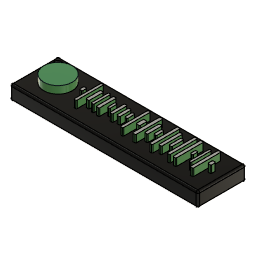
Spotify_Bars v3 (Autodesk Fusion 360 design; units mm, degrees)
Autodesk Fusion 360 part; units mm, degrees
sketch "Sketch1" plane through (0, 0, 0) normal (0, 0, 1) x (1, 0, 0)
  line L0 (0, 0) -> (50.8, 0)
  line L1 (50.8, 0) -> (50.8, 13.0624)
  line L2 (50.8, 13.0624) -> (0, 13.0624)
  line L3 (0, 13.0624) -> (0, 0)
  dimension "d1" = 50.8
  constraint horizontal L0
  constraint vertical L1
  constraint horizontal L2
  constraint vertical L3
  constraint coincident L0.start L3.end
  measures "d1" distance of L0.start L0.end
extrude "Extrude1" add sketch "Sketch1" along normal blind 4
sketch "Sketch2" plane through (0, 0, 4) normal (0, 0, 1) x (-1, 0, 0)
  line L0 (0, -13.0624) -> (0, 0)
  line L1 (0, 0) -> (-50.8, 0)
  line L2 (-50.8, 0) -> (-50.8, -13.0624)
  line L3 (-50.8, -13.0624) -> (0, -13.0624)
  line L4 (-12.7231, -7.3007) -> (-13.5424, -7.3007)
  line L5 (-13.5424, -7.3007) -> (-13.5424, -6.0226)
  line L6 (-13.5424, -6.0226) -> (-12.7231, -6.0226)
  line L7 (-12.7231, -6.0226) -> (-12.7231, -7.3007)
  constraint horizontal L4
  constraint vertical L5
  constraint horizontal L6
  constraint vertical L7
extrude "Extrude2" add sketch "Sketch2" along normal blind 2 contours L4 L5 L6 L7
sketch "Sketch3" plane through (0, 0, 4) normal (0, 0, 1) x (-1, 0, 0)
  line L0 (-12.7231, -6.0226) -> (-12.7231, -7.3007)
  line L1 (-12.7231, -7.3007) -> (-13.5424, -7.3007)
  line L2 (-13.5424, -7.3007) -> (-13.5424, -6.0226)
  line L3 (-13.5424, -6.0226) -> (-12.7231, -6.0226)
  line L4 (0, -13.0624) -> (0, 0)
  line L5 (0, 0) -> (-50.8, 0)
  line L6 (-50.8, 0) -> (-50.8, -13.0624)
  line L7 (-50.8, -13.0624) -> (0, -13.0624)
  line L8 (-14.2857, -10.434) -> (-15, -10.434)
  line L9 (-15, -10.434) -> (-15, -3)
  line L10 (-15, -3) -> (-14.2857, -3)
  line L11 (-14.2857, -3) -> (-14.2857, -10.434)
  constraint horizontal L8
  constraint vertical L9
  constraint horizontal L10
  constraint vertical L11
extrude "Extrude3" add sketch "Sketch3" along normal blind 2 contours L8 L9 L10 L11
sketch "Sketch4" plane through (0, 0, 4) normal (0, 0, 1) x (-1, 0, 0)
  line L0 (-14.2857, -3) -> (-14.2857, -10.434)
  line L1 (-14.2857, -10.434) -> (-15, -10.434)
  line L2 (-15, -10.434) -> (-15, -3)
  line L3 (-15, -3) -> (-14.2857, -3)
  line L4 (-12.7231, -6.0226) -> (-12.7231, -7.3007)
  line L5 (-12.7231, -7.3007) -> (-13.5424, -7.3007)
  line L6 (-13.5424, -7.3007) -> (-13.5424, -6.0226)
  line L7 (-13.5424, -6.0226) -> (-12.7231, -6.0226)
  line L8 (0, -13.0624) -> (0, 0)
  line L9 (0, 0) -> (-50.8, 0)
  line L10 (-50.8, 0) -> (-50.8, -13.0624)
  line L11 (-50.8, -13.0624) -> (0, -13.0624)
  line L12 (-15.8233, -8.6464) -> (-16.7081, -8.6464)
  line L13 (-16.7081, -8.6464) -> (-16.7081, -4.681)
  line L14 (-16.7081, -4.681) -> (-15.8233, -4.681)
  line L15 (-15.8233, -4.681) -> (-15.8233, -8.6464)
  constraint horizontal L12
  constraint vertical L13
  constraint horizontal L14
  constraint vertical L15
extrude "Extrude4" add sketch "Sketch4" along normal blind 2 contours L12 L13 L14 L15
sketch "Sketch5" plane through (0, 0, 4) normal (0, 0, 1) x (-1, 0, 0)
  line L0 (-15.8233, -4.681) -> (-15.8233, -8.6464)
  line L1 (-15.8233, -8.6464) -> (-16.7081, -8.6464)
  line L2 (-16.7081, -8.6464) -> (-16.7081, -4.681)
  line L3 (-16.7081, -4.681) -> (-15.8233, -4.681)
  line L4 (-14.2857, -3) -> (-14.2857, -10.434)
  line L5 (-14.2857, -10.434) -> (-15, -10.434)
  line L6 (-15, -10.434) -> (-15, -3)
  line L7 (-15, -3) -> (-14.2857, -3)
  line L8 (-12.7231, -6.0226) -> (-12.7231, -7.3007)
  line L9 (-12.7231, -7.3007) -> (-13.5424, -7.3007)
  line L10 (-13.5424, -7.3007) -> (-13.5424, -6.0226)
  line L11 (-13.5424, -6.0226) -> (-12.7231, -6.0226)
  line L12 (0, -13.0624) -> (0, 0)
  line L13 (0, 0) -> (-50.8, 0)
  line L14 (-50.8, 0) -> (-50.8, -13.0624)
  line L15 (-50.8, -13.0624) -> (0, -13.0624)
  line L16 (-17.5123, -9.1117) -> (-18.2005, -9.1117)
  line L17 (-18.2005, -9.1117) -> (-18.2005, -4.3925)
  line L18 (-18.2005, -4.3925) -> (-17.5123, -4.3925)
  line L19 (-17.5123, -4.3925) -> (-17.5123, -9.1117)
  constraint horizontal L16
  constraint vertical L17
  constraint horizontal L18
  constraint vertical L19
extrude "Extrude5" add sketch "Sketch5" along normal blind 2 contours L16 L17 L18 L19
sketch "Sketch6" plane through (0, 0, 4) normal (0, 0, 1) x (-1, 0, 0)
  line L0 (-17.5123, -4.3925) -> (-17.5123, -9.1117)
  line L1 (-17.5123, -9.1117) -> (-18.2005, -9.1117)
  line L2 (-18.2005, -9.1117) -> (-18.2005, -4.3925)
  line L3 (-18.2005, -4.3925) -> (-17.5123, -4.3925)
  line L4 (-15.8233, -4.681) -> (-15.8233, -8.6464)
  line L5 (-15.8233, -8.6464) -> (-16.7081, -8.6464)
  line L6 (-16.7081, -8.6464) -> (-16.7081, -4.681)
  line L7 (-16.7081, -4.681) -> (-15.8233, -4.681)
  line L8 (-14.2857, -3) -> (-14.2857, -10.434)
  line L9 (-14.2857, -10.434) -> (-15, -10.434)
  line L10 (-15, -10.434) -> (-15, -3)
  line L11 (-15, -3) -> (-14.2857, -3)
  line L12 (-12.7231, -6.0226) -> (-12.7231, -7.3007)
  line L13 (-12.7231, -7.3007) -> (-13.5424, -7.3007)
  line L14 (-13.5424, -7.3007) -> (-13.5424, -6.0226)
  line L15 (-13.5424, -6.0226) -> (-12.7231, -6.0226)
  line L16 (0, -13.0624) -> (0, 0)
  line L17 (0, 0) -> (-50.8, 0)
  line L18 (-50.8, 0) -> (-50.8, -13.0624)
  line L19 (-50.8, -13.0624) -> (0, -13.0624)
  line L20 (-19, -9) -> (-19.8456, -9)
  line L21 (-19.8456, -9) -> (-19.8456, -4.261)
  line L22 (-19.8456, -4.261) -> (-19, -4.261)
  line L23 (-19, -4.261) -> (-19, -9)
  line L24 (-20.6977, -7.7349) -> (-21.3531, -7.7349)
  line L25 (-21.3531, -7.7349) -> (-21.3531, -5.6047)
  line L26 (-21.3531, -5.6047) -> (-20.6977, -5.6047)
  line L27 (-20.6977, -5.6047) -> (-20.6977, -7.7349)
  line L28 (-22.2708, -8.718) -> (-23.0573, -8.718)
  line L29 (-23.0573, -8.718) -> (-23.0573, -4.687)
  line L30 (-23.0573, -4.687) -> (-22.2708, -4.687)
  line L31 (-22.2708, -4.687) -> (-22.2708, -8.718)
  line L32 (-23.8111, -8.2592) -> (-24.6304, -8.2592)
  line L33 (-24.6304, -8.2592) -> (-24.6304, -5.0475)
  line L34 (-24.6304, -5.0475) -> (-23.8111, -5.0475)
  line L35 (-23.8111, -5.0475) -> (-23.8111, -8.2592)
  line L36 (-25.3514, -7.7349) -> (-26.1051, -7.7349)
  line L37 (-26.1051, -7.7349) -> (-26.1051, -5.6374)
  line L38 (-26.1051, -5.6374) -> (-25.3514, -5.6374)
  line L39 (-25.3514, -5.6374) -> (-25.3514, -7.7349)
  line L40 (-26.9572, -10.3567) -> (-27.711, -10.3567)
  line L41 (-27.711, -10.3567) -> (-27.711, -2.8845)
  line L42 (-27.711, -2.8845) -> (-26.9572, -2.8845)
  line L43 (-26.9572, -2.8845) -> (-26.9572, -10.3567)
  line L44 (-28.432, -7.7021) -> (-29.4479, -7.7021)
  line L45 (-29.4479, -7.7021) -> (-29.4479, -5.6374)
  line L46 (-29.4479, -5.6374) -> (-28.432, -5.6374)
  line L47 (-28.432, -5.6374) -> (-28.432, -7.7021)
  line L48 (-30.1034, -10.3894) -> (-31, -10.3894)
  line L49 (-31, -10.3894) -> (-31, -3)
  line L50 (-31, -3) -> (-30.1034, -3)
  line L51 (-30.1034, -3) -> (-30.1034, -10.3894)
  line L52 (-31.6437, -8.718) -> (-32.4957, -8.718)
  line L53 (-32.4957, -8.718) -> (-32.4957, -4.687)
  line L54 (-32.4957, -4.687) -> (-31.6437, -4.687)
  line L55 (-31.6437, -4.687) -> (-31.6437, -8.718)
  line L56 (-33.2495, -7.7349) -> (-34.0033, -7.7349)
  line L57 (-34.0033, -7.7349) -> (-34.0033, -5.5719)
  line L58 (-34.0033, -5.5719) -> (-33.2495, -5.5719)
  line L59 (-33.2495, -5.5719) -> (-33.2495, -7.7349)
  line L60 (-34.7898, -10.4877) -> (-35.6091, -10.4877)
  line L61 (-35.6091, -10.4877) -> (-35.6091, -2.8845)
  line L62 (-35.6091, -2.8845) -> (-34.7898, -2.8845)
  line L63 (-34.7898, -2.8845) -> (-34.7898, -10.4877)
  line L64 (-36.3957, -9.5373) -> (-37.215, -9.5373)
  line L65 (-37.215, -9.5373) -> (-37.215, -3.7694)
  line L66 (-37.215, -3.7694) -> (-36.3957, -3.7694)
  line L67 (-36.3957, -3.7694) -> (-36.3957, -9.5373)
  line L68 (-37.9032, -8.3575) -> (-38.6897, -8.3575)
  line L69 (-38.6897, -8.3575) -> (-38.6897, -5.0475)
  line L70 (-38.6897, -5.0475) -> (-37.9032, -5.0475)
  line L71 (-37.9032, -5.0475) -> (-37.9032, -8.3575)
  line L72 (-39.509, -10.455) -> (-40.2956, -10.455)
  line L73 (-40.2956, -10.455) -> (-40.2956, -2.9501)
  line L74 (-40.2956, -2.9501) -> (-39.509, -2.9501)
  line L75 (-39.509, -2.9501) -> (-39.509, -10.455)
  line L76 (-41.0821, -10.455) -> (-41.9342, -10.455)
  line L77 (-41.9342, -10.455) -> (-41.9342, -2.9501)
  line L78 (-41.9342, -2.9501) -> (-41.0821, -2.9501)
  line L79 (-41.0821, -2.9501) -> (-41.0821, -10.455)
  line L80 (-42.7535, -7.4399) -> (-43.4417, -7.4399)
  line L81 (-43.4417, -7.4399) -> (-43.4417, -5.9979)
  line L82 (-43.4417, -5.9979) -> (-42.7535, -5.9979)
  line L83 (-42.7535, -5.9979) -> (-42.7535, -7.4399)
  line L84 (-44.3594, -9.5701) -> (-45, -9.5701)
  line L85 (-45, -9.5701) -> (-45, -4)
  line L86 (-45, -4) -> (-44.3594, -4)
  line L87 (-44.3594, -4) -> (-44.3594, -9.5701)
  line L88 (-45.8669, -10.4877) -> (-46.6534, -10.4877)
  line L89 (-46.6534, -10.4877) -> (-46.6534, -2.9501)
  line L90 (-46.6534, -2.9501) -> (-45.8669, -2.9501)
  line L91 (-45.8669, -2.9501) -> (-45.8669, -10.4877)
  line L92 (-47.44, -7.3744) -> (-48.2921, -7.3744)
  line L93 (-48.2921, -7.3744) -> (-48.2921, -5.9979)
  line L94 (-48.2921, -5.9979) -> (-47.44, -5.9979)
  line L95 (-47.44, -5.9979) -> (-47.44, -7.3744)
  constraint horizontal L20
  constraint vertical L21
  constraint horizontal L22
  constraint vertical L23
  constraint horizontal L24
  constraint vertical L25
  constraint horizontal L26
  constraint vertical L27
  constraint horizontal L28
  constraint vertical L29
  constraint horizontal L30
  constraint vertical L31
  constraint horizontal L32
  constraint vertical L33
  constraint horizontal L34
  constraint vertical L35
  constraint horizontal L36
  constraint vertical L37
  constraint horizontal L38
  constraint vertical L39
  constraint horizontal L40
  constraint vertical L41
  constraint horizontal L42
  constraint vertical L43
  constraint horizontal L44
  constraint vertical L45
  constraint horizontal L46
  constraint vertical L47
  constraint horizontal L48
  constraint vertical L49
  constraint horizontal L50
  constraint vertical L51
  constraint horizontal L52
  constraint vertical L53
  constraint horizontal L54
  constraint vertical L55
  constraint horizontal L56
  constraint vertical L57
  constraint horizontal L58
  constraint vertical L59
  constraint horizontal L60
  constraint vertical L61
  constraint horizontal L62
  constraint vertical L63
  constraint horizontal L64
  constraint vertical L65
  constraint horizontal L66
  constraint vertical L67
  constraint horizontal L68
  constraint vertical L69
  constraint horizontal L70
  constraint vertical L71
  constraint horizontal L72
  constraint vertical L73
  constraint horizontal L74
  constraint vertical L75
  constraint horizontal L76
  constraint vertical L77
  constraint horizontal L78
  constraint vertical L79
  constraint horizontal L80
  constraint vertical L81
  constraint horizontal L82
  constraint vertical L83
  constraint horizontal L84
  constraint vertical L85
  constraint horizontal L86
  constraint vertical L87
  constraint horizontal L88
  constraint vertical L89
  constraint horizontal L90
  constraint vertical L91
  constraint horizontal L92
  constraint vertical L93
  constraint horizontal L94
  constraint vertical L95
extrude "Extrude6" add sketch "Sketch6" along normal blind 2 contours L20 L21 L22 L23 | L24 L25 L26 L27 | L28 L29 L30 L31 | L32 L33 L34 L35 | L36 L37 L38 L39 | L40 L41 L42 L43 | L44 L45 L46 L47 | L48 L49 L50 L51 | L52 L53 L54 L55 | L56 L57 L58 L59 | L60 L61 L62 L63 | L64 L65 L66 L67 | L68 L69 L70 L71 | L72 L73 L74 L75 | L76 L77 L78 L79 | L80 L81 L82 L83 | L84 L85 L86 L87
sketch "Sketch7" plane through (0, 0, 4) normal (0, 0, 1) x (-1, 0, 0)
  line L0 (-19, -4.261) -> (-19, -9)
  line L1 (-19, -9) -> (-19.8456, -9)
  line L2 (-19.8456, -9) -> (-19.8456, -4.261)
  line L3 (-19.8456, -4.261) -> (-19, -4.261)
  line L4 (-25.3514, -5.6374) -> (-25.3514, -7.7349)
  line L5 (-25.3514, -7.7349) -> (-26.1051, -7.7349)
  line L6 (-26.1051, -7.7349) -> (-26.1051, -5.6374)
  line L7 (-26.1051, -5.6374) -> (-25.3514, -5.6374)
  line L8 (-31.6437, -4.687) -> (-31.6437, -8.718)
  line L9 (-31.6437, -8.718) -> (-32.4957, -8.718)
  line L10 (-32.4957, -8.718) -> (-32.4957, -4.687)
  line L11 (-32.4957, -4.687) -> (-31.6437, -4.687)
  line L12 (-37.9032, -5.0475) -> (-37.9032, -8.3575)
  line L13 (-37.9032, -8.3575) -> (-38.6897, -8.3575)
  line L14 (-38.6897, -8.3575) -> (-38.6897, -5.0475)
  line L15 (-38.6897, -5.0475) -> (-37.9032, -5.0475)
  line L16 (-44.3594, -4) -> (-44.3594, -9.5701)
  line L17 (-44.3594, -9.5701) -> (-45, -9.5701)
  line L18 (-45, -9.5701) -> (-45, -4)
  line L19 (-45, -4) -> (-44.3594, -4)
  line L20 (-39.509, -2.9501) -> (-39.509, -10.455)
  line L21 (-39.509, -10.455) -> (-40.2956, -10.455)
  line L22 (-40.2956, -10.455) -> (-40.2956, -2.9501)
  line L23 (-40.2956, -2.9501) -> (-39.509, -2.9501)
  line L24 (-33.2495, -5.5719) -> (-33.2495, -7.7349)
  line L25 (-33.2495, -7.7349) -> (-34.0033, -7.7349)
  line L26 (-34.0033, -7.7349) -> (-34.0033, -5.5719)
  line L27 (-34.0033, -5.5719) -> (-33.2495, -5.5719)
  line L28 (-26.9572, -2.8845) -> (-26.9572, -10.3567)
  line L29 (-26.9572, -10.3567) -> (-27.711, -10.3567)
  line L30 (-27.711, -10.3567) -> (-27.711, -2.8845)
  line L31 (-27.711, -2.8845) -> (-26.9572, -2.8845)
  line L32 (-20.6977, -5.6047) -> (-20.6977, -7.7349)
  line L33 (-20.6977, -7.7349) -> (-21.3531, -7.7349)
  line L34 (-21.3531, -7.7349) -> (-21.3531, -5.6047)
  line L35 (-21.3531, -5.6047) -> (-20.6977, -5.6047)
  line L36 (-23.8111, -5.0475) -> (-23.8111, -8.2592)
  line L37 (-23.8111, -8.2592) -> (-24.6304, -8.2592)
  line L38 (-24.6304, -8.2592) -> (-24.6304, -5.0475)
  line L39 (-24.6304, -5.0475) -> (-23.8111, -5.0475)
  line L40 (-30.1034, -3) -> (-30.1034, -10.3894)
  line L41 (-30.1034, -10.3894) -> (-31, -10.3894)
  line L42 (-31, -10.3894) -> (-31, -3)
  line L43 (-31, -3) -> (-30.1034, -3)
  line L44 (-36.3957, -3.7694) -> (-36.3957, -9.5373)
  line L45 (-36.3957, -9.5373) -> (-37.215, -9.5373)
  line L46 (-37.215, -9.5373) -> (-37.215, -3.7694)
  line L47 (-37.215, -3.7694) -> (-36.3957, -3.7694)
  line L48 (-42.7535, -5.9979) -> (-42.7535, -7.4399)
  line L49 (-42.7535, -7.4399) -> (-43.4417, -7.4399)
  line L50 (-43.4417, -7.4399) -> (-43.4417, -5.9979)
  line L51 (-43.4417, -5.9979) -> (-42.7535, -5.9979)
  line L52 (-41.0821, -2.9501) -> (-41.0821, -10.455)
  line L53 (-41.0821, -10.455) -> (-41.9342, -10.455)
  line L54 (-41.9342, -10.455) -> (-41.9342, -2.9501)
  line L55 (-41.9342, -2.9501) -> (-41.0821, -2.9501)
  line L56 (-34.7898, -2.8845) -> (-34.7898, -10.4877)
  line L57 (-34.7898, -10.4877) -> (-35.6091, -10.4877)
  line L58 (-35.6091, -10.4877) -> (-35.6091, -2.8845)
  line L59 (-35.6091, -2.8845) -> (-34.7898, -2.8845)
  line L60 (-28.432, -5.6374) -> (-28.432, -7.7021)
  line L61 (-28.432, -7.7021) -> (-29.4479, -7.7021)
  line L62 (-29.4479, -7.7021) -> (-29.4479, -5.6374)
  line L63 (-29.4479, -5.6374) -> (-28.432, -5.6374)
  line L64 (-22.2708, -4.687) -> (-22.2708, -8.718)
  line L65 (-22.2708, -8.718) -> (-23.0573, -8.718)
  line L66 (-23.0573, -8.718) -> (-23.0573, -4.687)
  line L67 (-23.0573, -4.687) -> (-22.2708, -4.687)
  line L68 (-17.5123, -4.3925) -> (-17.5123, -9.1117)
  line L69 (-17.5123, -9.1117) -> (-18.2005, -9.1117)
  line L70 (-18.2005, -9.1117) -> (-18.2005, -4.3925)
  line L71 (-18.2005, -4.3925) -> (-17.5123, -4.3925)
  line L72 (-15.8233, -4.681) -> (-15.8233, -8.6464)
  line L73 (-15.8233, -8.6464) -> (-16.7081, -8.6464)
  line L74 (-16.7081, -8.6464) -> (-16.7081, -4.681)
  line L75 (-16.7081, -4.681) -> (-15.8233, -4.681)
  line L76 (-14.2857, -3) -> (-14.2857, -10.434)
  line L77 (-14.2857, -10.434) -> (-15, -10.434)
  line L78 (-15, -10.434) -> (-15, -3)
  line L79 (-15, -3) -> (-14.2857, -3)
  line L80 (-12.7231, -6.0226) -> (-12.7231, -7.3007)
  line L81 (-12.7231, -7.3007) -> (-13.5424, -7.3007)
  line L82 (-13.5424, -7.3007) -> (-13.5424, -6.0226)
  line L83 (-13.5424, -6.0226) -> (-12.7231, -6.0226)
  line L84 (0, -13.0624) -> (0, 0)
  line L85 (0, 0) -> (-50.8, 0)
  line L86 (-50.8, 0) -> (-50.8, -13.0624)
  line L87 (-50.8, -13.0624) -> (0, -13.0624)
  line L88 (-45.7946, -10.487) -> (-46.614, -10.487)
  line L89 (-46.614, -10.487) -> (-46.614, -2.8838)
  line L90 (-46.614, -2.8838) -> (-45.7946, -2.8838)
  line L91 (-45.7946, -2.8838) -> (-45.7946, -10.487)
  line L92 (-47.4333, -7.3408) -> (-48.3181, -7.3408)
  line L93 (-48.3181, -7.3408) -> (-48.3181, -6.0299)
  line L94 (-48.3181, -6.0299) -> (-47.4333, -6.0299)
  line L95 (-47.4333, -6.0299) -> (-47.4333, -7.3408)
  constraint horizontal L88
  constraint vertical L89
  constraint horizontal L90
  constraint vertical L91
  constraint horizontal L92
  constraint vertical L93
  constraint horizontal L94
  constraint vertical L95
extrude "Extrude7" add sketch "Sketch7" along normal blind 2 contours L88 L89 L90 L91 | L92 L93 L94 L95
fillet "Fillet1" radius 0.2 3 edges at (12.7231, 6.0226, 5) (12.7231, 7.3007, 5) (13.5424, 6.0226, 5)
fillet "Fillet2" radius 0.2 45 edges at (14.2857, 10.434, 5) (15, 10.434, 5) (15, 3, 5) (15.8233, 8.6464, 5) (16.7081, 8.6464, 5) (17.5123, 9.1117, 5) (16.7081, 4.681, 5) (15.8233, 4.681, 5) (14.2857, 3, 5) (13.5424, 7.3007, 5) (17.5123, 4.3925, 5) (18.2005, 9.1117, 5) (18.2005, 4.3925, 5) (19, 9, 5) (19.8456, 9, 5) (19, 4.261, 5) (19.8456, 4.261, 5) (20.6977, 7.7349, 5) (20.6977, 5.6047, 5) (21.3531, 7.7349, 5) (21.3531, 5.6047, 5) (22.2708, 8.718, 5) (23.0573, 8.718, 5) (22.2708, 4.687, 5) (23.0573, 4.687, 5) (23.8111, 8.2592, 5) (23.8111, 5.0475, 5) (24.6304, 8.2592, 5) (24.6304, 5.0475, 5) (25.3514, 7.7349, 5) (25.3514, 5.6374, 5) (26.1051, 7.7349, 5) (26.1051, 5.6374, 5) (26.9572, 10.3567, 5) (27.711, 10.3567, 5) (26.9572, 2.8845, 5) (27.711, 2.8845, 5) (28.432, 7.7021, 5) (28.432, 5.6374, 5) (29.4479, 7.7021, 5) (29.4479, 5.6374, 5) (30.1034, 10.3894, 5) (30.1034, 3, 5) (31, 10.3894, 5) (31.6437, 8.718, 5)
fillet "Fillet3" radius 0.2 44 edges at (31.6437, 4.687, 5) (31, 3, 5) (32.4957, 4.687, 5) (32.4957, 8.718, 5) (33.2495, 5.5719, 5) (33.2495, 7.7349, 5) (34.0033, 7.7349, 5) (34.0033, 5.5719, 5) (34.7898, 10.4877, 5) (35.6091, 10.4877, 5) (34.7898, 2.8845, 5) (35.6091, 2.8845, 5) (36.3957, 9.5373, 5) (36.3957, 3.7694, 5) (37.215, 9.5373, 5) (37.215, 3.7694, 5) (37.9032, 8.3575, 5) (37.9032, 5.0475, 5) (38.6897, 8.3575, 5) (38.6897, 5.0475, 5) (39.509, 10.455, 5) (39.509, 2.9501, 5) (40.2956, 10.455, 5) (40.2956, 2.9501, 5) (41.0821, 10.455, 5) (41.0821, 2.9501, 5) (41.9342, 10.455, 5) (41.9342, 2.9501, 5) (42.7535, 7.4399, 5) (42.7535, 5.9979, 5) (43.4417, 5.9979, 5) (43.4417, 7.4399, 5) (44.3594, 9.5701, 5) (45, 9.5701, 5) (44.3594, 4, 5) (45, 4, 5) (45.7946, 10.487, 5) (45.7946, 2.8838, 5) (46.614, 10.487, 5) (46.614, 2.8838, 5) (47.4333, 7.3408, 5) (47.4333, 6.0299, 5) (48.3181, 7.3408, 5) (48.3181, 6.0299, 5)
sketch "Sketch8" plane through (0, 0, 4) normal (0, 0, 1) x (-1, 0, 0)
  line L0 (-47.4333, -6.2299) -> (-47.4333, -7.1408)
  arc A0 (-47.6333, -7.3408) -> (-47.4333, -7.1408) centre (-47.6333, -7.1408) ccw
  line L1 (-47.6333, -7.3408) -> (-48.1181, -7.3408)
  arc A1 (-48.3181, -7.1408) -> (-48.1181, -7.3408) centre (-48.1181, -7.1408) ccw
  line L2 (-48.3181, -7.1408) -> (-48.3181, -6.2299)
  arc A2 (-48.1181, -6.0299) -> (-48.3181, -6.2299) centre (-48.1181, -6.2299) ccw
  line L3 (-48.1181, -6.0299) -> (-47.6333, -6.0299)
  arc A3 (-47.4333, -6.2299) -> (-47.6333, -6.0299) centre (-47.6333, -6.2299) ccw
  line L4 (-45.7946, -3.0838) -> (-45.7946, -10.287)
  arc A4 (-45.9946, -10.487) -> (-45.7946, -10.287) centre (-45.9946, -10.287) ccw
  line L5 (-45.9946, -10.487) -> (-46.414, -10.487)
  arc A5 (-46.614, -10.287) -> (-46.414, -10.487) centre (-46.414, -10.287) ccw
  line L6 (-46.614, -10.287) -> (-46.614, -3.0838)
  arc A6 (-46.414, -2.8838) -> (-46.614, -3.0838) centre (-46.414, -3.0838) ccw
  line L7 (-46.414, -2.8838) -> (-45.9946, -2.8838)
  arc A7 (-45.7946, -3.0838) -> (-45.9946, -2.8838) centre (-45.9946, -3.0838) ccw
  line L8 (-19, -4.461) -> (-19, -8.8)
  arc A8 (-19.2, -9) -> (-19, -8.8) centre (-19.2, -8.8) ccw
  line L9 (-19.2, -9) -> (-19.6456, -9)
  arc A9 (-19.8456, -8.8) -> (-19.6456, -9) centre (-19.6456, -8.8) ccw
  line L10 (-19.8456, -8.8) -> (-19.8456, -4.461)
  arc A10 (-19.6456, -4.261) -> (-19.8456, -4.461) centre (-19.6456, -4.461) ccw
  line L11 (-19.6456, -4.261) -> (-19.2, -4.261)
  arc A11 (-19, -4.461) -> (-19.2, -4.261) centre (-19.2, -4.461) ccw
  line L12 (-25.3514, -5.8374) -> (-25.3514, -7.5349)
  arc A12 (-25.5514, -7.7349) -> (-25.3514, -7.5349) centre (-25.5514, -7.5349) ccw
  line L13 (-25.5514, -7.7349) -> (-25.9051, -7.7349)
  arc A13 (-26.1051, -7.5349) -> (-25.9051, -7.7349) centre (-25.9051, -7.5349) ccw
  line L14 (-26.1051, -7.5349) -> (-26.1051, -5.8374)
  arc A14 (-25.9051, -5.6374) -> (-26.1051, -5.8374) centre (-25.9051, -5.8374) ccw
  line L15 (-25.9051, -5.6374) -> (-25.5514, -5.6374)
  arc A15 (-25.3514, -5.8374) -> (-25.5514, -5.6374) centre (-25.5514, -5.8374) ccw
  line L16 (-31.6437, -4.887) -> (-31.6437, -8.518)
  arc A16 (-31.8437, -8.718) -> (-31.6437, -8.518) centre (-31.8437, -8.518) ccw
  line L17 (-31.8437, -8.718) -> (-32.2957, -8.718)
  arc A17 (-32.4957, -8.518) -> (-32.2957, -8.718) centre (-32.2957, -8.518) ccw
  line L18 (-32.4957, -8.518) -> (-32.4957, -4.887)
  arc A18 (-32.2957, -4.687) -> (-32.4957, -4.887) centre (-32.2957, -4.887) ccw
  line L19 (-32.2957, -4.687) -> (-31.8437, -4.687)
  arc A19 (-31.6437, -4.887) -> (-31.8437, -4.687) centre (-31.8437, -4.887) ccw
  line L20 (-37.9032, -5.2475) -> (-37.9032, -8.1575)
  arc A20 (-38.1032, -8.3575) -> (-37.9032, -8.1575) centre (-38.1032, -8.1575) ccw
  line L21 (-38.1032, -8.3575) -> (-38.4897, -8.3575)
  arc A21 (-38.6897, -8.1575) -> (-38.4897, -8.3575) centre (-38.4897, -8.1575) ccw
  line L22 (-38.6897, -8.1575) -> (-38.6897, -5.2475)
  arc A22 (-38.4897, -5.0475) -> (-38.6897, -5.2475) centre (-38.4897, -5.2475) ccw
  line L23 (-38.4897, -5.0475) -> (-38.1032, -5.0475)
  arc A23 (-37.9032, -5.2475) -> (-38.1032, -5.0475) centre (-38.1032, -5.2475) ccw
  line L24 (-44.3594, -4.2) -> (-44.3594, -9.3701)
  arc A24 (-44.5594, -9.5701) -> (-44.3594, -9.3701) centre (-44.5594, -9.3701) ccw
  line L25 (-44.5594, -9.5701) -> (-44.8, -9.5701)
  arc A25 (-45, -9.3701) -> (-44.8, -9.5701) centre (-44.8, -9.3701) ccw
  line L26 (-45, -9.3701) -> (-45, -4.2)
  arc A26 (-44.8, -4) -> (-45, -4.2) centre (-44.8, -4.2) ccw
  line L27 (-44.8, -4) -> (-44.5594, -4)
  arc A27 (-44.3594, -4.2) -> (-44.5594, -4) centre (-44.5594, -4.2) ccw
  line L28 (-39.509, -3.1501) -> (-39.509, -10.255)
  arc A28 (-39.709, -10.455) -> (-39.509, -10.255) centre (-39.709, -10.255) ccw
  line L29 (-39.709, -10.455) -> (-40.0956, -10.455)
  arc A29 (-40.2956, -10.255) -> (-40.0956, -10.455) centre (-40.0956, -10.255) ccw
  line L30 (-40.2956, -10.255) -> (-40.2956, -3.1501)
  arc A30 (-40.0956, -2.9501) -> (-40.2956, -3.1501) centre (-40.0956, -3.1501) ccw
  line L31 (-40.0956, -2.9501) -> (-39.709, -2.9501)
  arc A31 (-39.509, -3.1501) -> (-39.709, -2.9501) centre (-39.709, -3.1501) ccw
  line L32 (-33.2495, -5.7719) -> (-33.2495, -7.5349)
  arc A32 (-33.4495, -7.7349) -> (-33.2495, -7.5349) centre (-33.4495, -7.5349) ccw
  line L33 (-33.4495, -7.7349) -> (-33.8033, -7.7349)
  arc A33 (-34.0033, -7.5349) -> (-33.8033, -7.7349) centre (-33.8033, -7.5349) ccw
  line L34 (-34.0033, -7.5349) -> (-34.0033, -5.7719)
  arc A34 (-33.8033, -5.5719) -> (-34.0033, -5.7719) centre (-33.8033, -5.7719) ccw
  line L35 (-33.8033, -5.5719) -> (-33.4495, -5.5719)
  arc A35 (-33.2495, -5.7719) -> (-33.4495, -5.5719) centre (-33.4495, -5.7719) ccw
  line L36 (-26.9572, -3.0845) -> (-26.9572, -10.1567)
  arc A36 (-27.1572, -10.3567) -> (-26.9572, -10.1567) centre (-27.1572, -10.1567) ccw
  line L37 (-27.1572, -10.3567) -> (-27.511, -10.3567)
  arc A37 (-27.711, -10.1567) -> (-27.511, -10.3567) centre (-27.511, -10.1567) ccw
  line L38 (-27.711, -10.1567) -> (-27.711, -3.0845)
  arc A38 (-27.511, -2.8845) -> (-27.711, -3.0845) centre (-27.511, -3.0845) ccw
  line L39 (-27.511, -2.8845) -> (-27.1572, -2.8845)
  arc A39 (-26.9572, -3.0845) -> (-27.1572, -2.8845) centre (-27.1572, -3.0845) ccw
  line L40 (-20.6977, -5.8047) -> (-20.6977, -7.5349)
  arc A40 (-20.8977, -7.7349) -> (-20.6977, -7.5349) centre (-20.8977, -7.5349) ccw
  line L41 (-20.8977, -7.7349) -> (-21.1531, -7.7349)
  arc A41 (-21.3531, -7.5349) -> (-21.1531, -7.7349) centre (-21.1531, -7.5349) ccw
  line L42 (-21.3531, -7.5349) -> (-21.3531, -5.8047)
  arc A42 (-21.1531, -5.6047) -> (-21.3531, -5.8047) centre (-21.1531, -5.8047) ccw
  line L43 (-21.1531, -5.6047) -> (-20.8977, -5.6047)
  arc A43 (-20.6977, -5.8047) -> (-20.8977, -5.6047) centre (-20.8977, -5.8047) ccw
  line L44 (-23.8111, -5.2475) -> (-23.8111, -8.0592)
  arc A44 (-24.0111, -8.2592) -> (-23.8111, -8.0592) centre (-24.0111, -8.0592) ccw
  line L45 (-24.0111, -8.2592) -> (-24.4304, -8.2592)
  arc A45 (-24.6304, -8.0592) -> (-24.4304, -8.2592) centre (-24.4304, -8.0592) ccw
  line L46 (-24.6304, -8.0592) -> (-24.6304, -5.2475)
  arc A46 (-24.4304, -5.0475) -> (-24.6304, -5.2475) centre (-24.4304, -5.2475) ccw
  line L47 (-24.4304, -5.0475) -> (-24.0111, -5.0475)
  arc A47 (-23.8111, -5.2475) -> (-24.0111, -5.0475) centre (-24.0111, -5.2475) ccw
  line L48 (-30.1034, -3.2) -> (-30.1034, -10.1894)
  arc A48 (-30.3034, -10.3894) -> (-30.1034, -10.1894) centre (-30.3034, -10.1894) ccw
  line L49 (-30.3034, -10.3894) -> (-30.8, -10.3894)
  arc A49 (-31, -10.1894) -> (-30.8, -10.3894) centre (-30.8, -10.1894) ccw
  line L50 (-31, -10.1894) -> (-31, -3.2)
  arc A50 (-30.8, -3) -> (-31, -3.2) centre (-30.8, -3.2) ccw
  line L51 (-30.8, -3) -> (-30.3034, -3)
  arc A51 (-30.1034, -3.2) -> (-30.3034, -3) centre (-30.3034, -3.2) ccw
  line L52 (-36.3957, -3.9694) -> (-36.3957, -9.3373)
  arc A52 (-36.5957, -9.5373) -> (-36.3957, -9.3373) centre (-36.5957, -9.3373) ccw
  line L53 (-36.5957, -9.5373) -> (-37.015, -9.5373)
  arc A53 (-37.215, -9.3373) -> (-37.015, -9.5373) centre (-37.015, -9.3373) ccw
  line L54 (-37.215, -9.3373) -> (-37.215, -3.9694)
  arc A54 (-37.015, -3.7694) -> (-37.215, -3.9694) centre (-37.015, -3.9694) ccw
  line L55 (-37.015, -3.7694) -> (-36.5957, -3.7694)
  arc A55 (-36.3957, -3.9694) -> (-36.5957, -3.7694) centre (-36.5957, -3.9694) ccw
  line L56 (-42.7535, -6.1979) -> (-42.7535, -7.2399)
  arc A56 (-42.9535, -7.4399) -> (-42.7535, -7.2399) centre (-42.9535, -7.2399) ccw
  line L57 (-42.9535, -7.4399) -> (-43.2417, -7.4399)
  arc A57 (-43.4417, -7.2399) -> (-43.2417, -7.4399) centre (-43.2417, -7.2399) ccw
  line L58 (-43.4417, -7.2399) -> (-43.4417, -6.1979)
  arc A58 (-43.2417, -5.9979) -> (-43.4417, -6.1979) centre (-43.2417, -6.1979) ccw
  line L59 (-43.2417, -5.9979) -> (-42.9535, -5.9979)
  arc A59 (-42.7535, -6.1979) -> (-42.9535, -5.9979) centre (-42.9535, -6.1979) ccw
  line L60 (-41.0821, -3.1501) -> (-41.0821, -10.255)
  arc A60 (-41.2821, -10.455) -> (-41.0821, -10.255) centre (-41.2821, -10.255) ccw
  line L61 (-41.2821, -10.455) -> (-41.7342, -10.455)
  arc A61 (-41.9342, -10.255) -> (-41.7342, -10.455) centre (-41.7342, -10.255) ccw
  line L62 (-41.9342, -10.255) -> (-41.9342, -3.1501)
  arc A62 (-41.7342, -2.9501) -> (-41.9342, -3.1501) centre (-41.7342, -3.1501) ccw
  line L63 (-41.7342, -2.9501) -> (-41.2821, -2.9501)
  arc A63 (-41.0821, -3.1501) -> (-41.2821, -2.9501) centre (-41.2821, -3.1501) ccw
  line L64 (-34.7898, -3.0845) -> (-34.7898, -10.2877)
  arc A64 (-34.9898, -10.4877) -> (-34.7898, -10.2877) centre (-34.9898, -10.2877) ccw
  line L65 (-34.9898, -10.4877) -> (-35.4091, -10.4877)
  arc A65 (-35.6091, -10.2877) -> (-35.4091, -10.4877) centre (-35.4091, -10.2877) ccw
  line L66 (-35.6091, -10.2877) -> (-35.6091, -3.0845)
  arc A66 (-35.4091, -2.8845) -> (-35.6091, -3.0845) centre (-35.4091, -3.0845) ccw
  line L67 (-35.4091, -2.8845) -> (-34.9898, -2.8845)
  arc A67 (-34.7898, -3.0845) -> (-34.9898, -2.8845) centre (-34.9898, -3.0845) ccw
  line L68 (-28.432, -5.8374) -> (-28.432, -7.5021)
  arc A68 (-28.632, -7.7021) -> (-28.432, -7.5021) centre (-28.632, -7.5021) ccw
  line L69 (-28.632, -7.7021) -> (-29.2479, -7.7021)
  arc A69 (-29.4479, -7.5021) -> (-29.2479, -7.7021) centre (-29.2479, -7.5021) ccw
  line L70 (-29.4479, -7.5021) -> (-29.4479, -5.8374)
  arc A70 (-29.2479, -5.6374) -> (-29.4479, -5.8374) centre (-29.2479, -5.8374) ccw
  line L71 (-29.2479, -5.6374) -> (-28.632, -5.6374)
  arc A71 (-28.432, -5.8374) -> (-28.632, -5.6374) centre (-28.632, -5.8374) ccw
  line L72 (-22.2708, -4.887) -> (-22.2708, -8.518)
  arc A72 (-22.4708, -8.718) -> (-22.2708, -8.518) centre (-22.4708, -8.518) ccw
  line L73 (-22.4708, -8.718) -> (-22.8573, -8.718)
  arc A73 (-23.0573, -8.518) -> (-22.8573, -8.718) centre (-22.8573, -8.518) ccw
  line L74 (-23.0573, -8.518) -> (-23.0573, -4.887)
  arc A74 (-22.8573, -4.687) -> (-23.0573, -4.887) centre (-22.8573, -4.887) ccw
  line L75 (-22.8573, -4.687) -> (-22.4708, -4.687)
  arc A75 (-22.2708, -4.887) -> (-22.4708, -4.687) centre (-22.4708, -4.887) ccw
  line L76 (-17.5123, -4.5925) -> (-17.5123, -8.9117)
  arc A76 (-17.7123, -9.1117) -> (-17.5123, -8.9117) centre (-17.7123, -8.9117) ccw
  line L77 (-17.7123, -9.1117) -> (-18.0005, -9.1117)
  arc A77 (-18.2005, -8.9117) -> (-18.0005, -9.1117) centre (-18.0005, -8.9117) ccw
  line L78 (-18.2005, -8.9117) -> (-18.2005, -4.5925)
  arc A78 (-18.0005, -4.3925) -> (-18.2005, -4.5925) centre (-18.0005, -4.5925) ccw
  line L79 (-18.0005, -4.3925) -> (-17.7123, -4.3925)
  arc A79 (-17.5123, -4.5925) -> (-17.7123, -4.3925) centre (-17.7123, -4.5925) ccw
  line L80 (-15.8233, -4.881) -> (-15.8233, -8.4464)
  arc A80 (-16.0233, -8.6464) -> (-15.8233, -8.4464) centre (-16.0233, -8.4464) ccw
  line L81 (-16.0233, -8.6464) -> (-16.5081, -8.6464)
  arc A81 (-16.7081, -8.4464) -> (-16.5081, -8.6464) centre (-16.5081, -8.4464) ccw
  line L82 (-16.7081, -8.4464) -> (-16.7081, -4.881)
  arc A82 (-16.5081, -4.681) -> (-16.7081, -4.881) centre (-16.5081, -4.881) ccw
  line L83 (-16.5081, -4.681) -> (-16.0233, -4.681)
  arc A83 (-15.8233, -4.881) -> (-16.0233, -4.681) centre (-16.0233, -4.881) ccw
  line L84 (-14.2857, -3.2) -> (-14.2857, -10.234)
  arc A84 (-14.4857, -10.434) -> (-14.2857, -10.234) centre (-14.4857, -10.234) ccw
  line L85 (-14.4857, -10.434) -> (-14.8, -10.434)
  arc A85 (-15, -10.234) -> (-14.8, -10.434) centre (-14.8, -10.234) ccw
  line L86 (-15, -10.234) -> (-15, -3.2)
  arc A86 (-14.8, -3) -> (-15, -3.2) centre (-14.8, -3.2) ccw
  line L87 (-14.8, -3) -> (-14.4857, -3)
  arc A87 (-14.2857, -3.2) -> (-14.4857, -3) centre (-14.4857, -3.2) ccw
  line L88 (-12.7231, -6.2226) -> (-12.7231, -7.1007)
  arc A88 (-12.9231, -7.3007) -> (-12.7231, -7.1007) centre (-12.9231, -7.1007) ccw
  line L89 (-12.9231, -7.3007) -> (-13.3424, -7.3007)
  arc A89 (-13.5424, -7.1007) -> (-13.3424, -7.3007) centre (-13.3424, -7.1007) ccw
  line L90 (-13.5424, -7.1007) -> (-13.5424, -6.2226)
  arc A90 (-13.3424, -6.0226) -> (-13.5424, -6.2226) centre (-13.3424, -6.2226) ccw
  line L91 (-13.3424, -6.0226) -> (-12.9231, -6.0226)
  arc A91 (-12.7231, -6.2226) -> (-12.9231, -6.0226) centre (-12.9231, -6.2226) ccw
  line L92 (0, -13.0624) -> (0, 0)
  line L93 (0, 0) -> (-50.8, 0)
  line L94 (-50.8, 0) -> (-50.8, -13.0624)
  line L95 (-50.8, -13.0624) -> (0, -13.0624)
  circle A92 centre (-6.2957, -6.7286) radius 3.8712
fillet "Fillet4" radius 0.5 6 edges at (25.4, 13.0624, 4) (0, 6.5312, 4) (25.4, 0, 4) (25.4, 0, 0) (0, 6.5312, 0) (25.4, 13.0624, 0)
fillet "Fillet5" radius 0.5 8 edges at (50.8, 13.0624, 2) (50.8, 12.9159, 0.1464) (50.8, 6.5312, 0) (50.8, 0.1464, 0.1464) (50.8, 0, 2) (50.8, 0.1464, 3.8536) (50.8, 6.5312, 4) (50.8, 12.9159, 3.8536)
fillet "Fillet6" radius 0.5 3 edges at (0.1464, 12.9159, 0.1464) (0, 13.0624, 2) (0.1464, 12.9159, 3.8536)
fillet "Fillet7" radius 0.5 3 edges at (0.1464, 0.1464, 0.1464) (0, 0, 2) (0.1464, 0.1464, 3.8536)
hole "Hole1" at (1.8136, 11.1543, 4) direction (0, 0, -1) diameter 2 depth 6 tip angle 118
extrude "Extrude8" add sketch "Sketch8" along normal blind 2 contours A92
sketch "Sketch11" plane through (0, 0, 6) normal (0, 0, 1) x (-1, 0, 0)
  circle A0 centre (-6.2957, -6.7286) radius 3.8712
